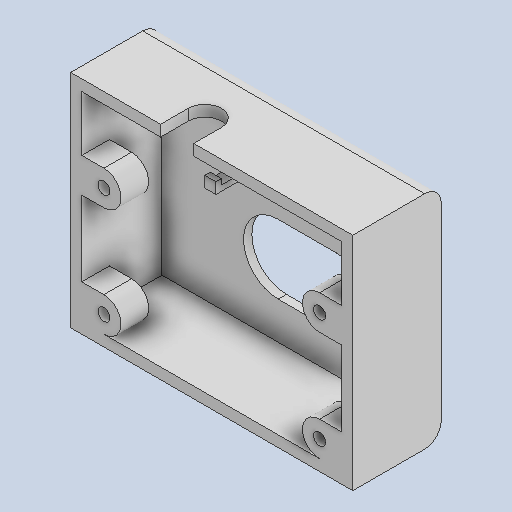
# Autodesk Inventor part: lidarhouse
Saved by Autodesk Inventor 2023.1 (Build 271208000, 208)
## iProperties
Created: 2023-03-22
Part Number: lidarhouse
Material: Generic
Document SubType Name: Modeling
Designer: liaar
Density: 1 g/cm^3
Appearance: Default
Author: liaar
Autodesk Inventor part; units mm, degrees
sketch "Sketch1" plane through (0, 0, 0) normal (0, 0, 1) x (1, 0, 0)
  line L0 (0, 0) -> (51, 0)
  line L1 (51, 0) -> (51, 40)
  line L2 (51, 40) -> (0, 40)
  line L3 (0, 40) -> (0, 0)
  dimension "d0" = 40
  dimension "d1" = 51
  constraints: 8 end point, 2 parallel, 1 horizontal, 1 perpendicular
  measures "d0" distance of L0.end L1.end
  measures "d1" distance of L1.end L2.end
extrude "Extrusion1" add sketch "Sketch1" along normal blind 16
sketch "Sketch2" plane through (0, 0, 16) normal (0, 0, 1) x (1, 0, 0)
  line L0 (2, 38) -> (49, 38)
  line L1 (49, 38) -> (49, 2)
  line L2 (49, 2) -> (2, 2)
  line L3 (2, 2) -> (2, 38)
  line L4 (51, 40) -> (0, 40) projected
  line L5 (0, 40) -> (0, 0) projected
  line L6 (51, 0) -> (51, 40) projected
  line L7 (0, 0) -> (51, 0) projected
  dimension "d4" = 2
  dimension "d5" = 2
  dimension "d6" = 2
  dimension "d7" = 2
  constraints: 8 end point, 2 parallel, 1 horizontal, 1 perpendicular
  measures "d4" distance between parallel lines of L4 L0
  measures "d5" distance between parallel lines of L5 L3
  measures "d6" distance between parallel lines of L6 L1
  measures "d7" distance between parallel lines of L7 L2
extrude "Extrusion2" cut sketch "Sketch2" against normal blind 14.5 contours L0 L1 L2 L3
fillet "Fillet1" radius 3 2 edges at (25.5, 40, 0) (25.5, 0, 0)
sketch "Sketch3" plane through (0, 0, 0) normal (0, 0, -1) x (-1, 0, 0)
  line L0 (-51, 3) -> (-51, 37) projected
  line L1 (0, 37) -> (0, 3) projected
  line L2 (-51, 37) -> (0, 37) projected
  line L3 (0, 3) -> (-51, 3) projected
  circle A0 centre (-33.5, 15) radius 6.25
  circle A1 centre (-23, 15) radius 6.25
  line L4 (-33.5, 21.25) -> (-23, 21.25)
  line L5 (-33.5, 8.75) -> (-23, 8.75)
  line L6 (0, 40) -> (-51, 40) projected
  point P0 (0, 0)
  point P1 (-28.25, 21.25)
  dimension "d49" = 12.5
  dimension "d51" = 10.5
  dimension "d52" = 12.5
  dimension "d54" = 17.5
  dimension "d55" = 22.75
  dimension "d58" = 25
  constraints: 4 end point, 4 point on circle, 4 tangent, 2 centre point, 1 horizontal alignment, 1 midpoint
  measures "d49" diameter of A0
  measures "d51" distance of A0.centre A1.centre
  measures "d52" diameter of A1
  measures "d54" distance from line of L0 A0.centre
  measures "d55" distance from line of L0 point (-28.25, 21.25)
  measures "d58" distance from line of L6 A0.centre
extrude "Extrusion3" cut sketch "Sketch3" against normal blind 14 contours A0 A1 | L4 A1 A0 | A0 A1 L5 | A1 A0 | A0 A1
sketch "Sketch4" plane through (0, 40, 16) normal (0, 1, 0) x (1, 0, 0)
  line L0 (35.25, 0) -> (21.25, 0)
  line L1 (21.25, 0) -> (21.25, 8)
  line L2 (21.25, 8) -> (35.25, 8)
  line L3 (35.25, 8) -> (35.25, 0)
  line L4 (51, 0) -> (0, 0) projected
  line L5 (0, 13) -> (0, 0) projected
  line L6 (51, 13) -> (51, 0) projected
  point P0 (0, 16)
  dimension "d18" = 14
  dimension "d19" = 8
  dimension "d20" = 21.25
  dimension "d21" = 15.75
  constraints: 8 end point, 2 parallel, 1 collinear, 1 horizontal, 1 perpendicular
  measures "d18" distance of L0.start L0.end
  measures "d19" distance of L0.end L1.end
  measures "d20" distance between parallel lines of L5 L1
  measures "d21" distance between parallel lines of L6 L3
ref_plane "Work Plane1" through (0, 0, 16) normal (0, 0, 1) x (1, 0, 0)
sketch "Sketch5" plane through (0, 0, 16) normal (0, 0, 1) x (1, 0, 0)
  circle A0 centre (6, 24.9) radius 3.1
  line L0 (49, 38) -> (49, 2) projected
  line L1 (6, 28) -> (2, 28)
  line L2 (6, 21.8) -> (2, 21.8)
  circle A1 centre (6, 24.9) radius 1.1
  line L3 (2, 2) -> (2, 38) projected
  line L4 (25.5, 34) -> (25.5, 3) construction
  line L5 (0, 3) -> (51, 3) construction
  line L6 (2, 2) -> (2, 38) construction
  line L7 (49, 38) -> (49, 2) construction
  circle A2 centre (6, 5.1) radius 3.1
  line L8 (6, 2) -> (2, 2)
  line L9 (6, 8.2) -> (2, 8.2)
  circle A3 centre (6, 5.1) radius 1.1
  line L10 (2, 38) -> (2, 2)
  line L11 (2, 38) -> (2, 2) construction
  circle A4 centre (45, 24.9) radius 3.1
  line L12 (45, 28) -> (49, 28)
  line L13 (45, 21.8) -> (49, 21.8)
  circle A5 centre (45, 24.9) radius 1.1
  line L14 (49, 2) -> (49, 38)
  line L15 (51, 3) -> (0, 3) construction
  line L16 (49, 2) -> (49, 38) construction
  line L17 (49, 38) -> (49, 2)
  line L18 (49, 38) -> (49, 2) construction
  line L19 (45, 8.2) -> (49, 8.2)
  circle A6 centre (45, 5.1) radius 3.1
  line L20 (45, 2) -> (49, 2)
  circle A7 centre (45, 5.1) radius 1.1
  line L21 (2, 38) -> (49, 38) projected
  line L22 (49, 2) -> (2, 2) projected
  point P0 (0, 0)
  point P1 (4, 28)
  point P2 (4, 2)
  point P3 (47, 28)
  point P4 (47, 2)
  point P5 (49, 8.2)
  point P6 (2, 2)
  point P7 (2, 8.2)
  point P8 (25.5, 38)
  dimension "d28" = 6.2
  dimension "d30" = 4
  dimension "d31" = 2.2
  dimension "d61" = 19.8
  dimension "d62" = 6.2
  constraints: 32 end point, 20 symmetric about line, 9 point on line, 8 centre point, 8 point on circle, 4 coincident, 2 horizontal, 2 midpoint, 2 tangent, 1 collinear, 5 other
  measures "d28" diameter of A0
  measures "d30" distance of L1.start L1.end
  measures "d31" diameter of A1
  measures "d61" distance of A2.centre A0.centre
  measures "d62" diameter of A2
extrude "Extrusion5" add sketch "Sketch5" against normal blind 5 contours A0 | A0 L2 L3 L1 | L9 A2 L8 L3 | A2 | L0 L13 A4 L12 | A4 | A6 | A6 L19 L0 L20
sketch "Sketch6" plane through (0, 0, 11) normal (0, 0, -1) x (-1, 0, 0)
  circle A0 centre (-45, 24.9) radius 1.1 projected
  line L0 (-45, 22.5906) -> (-47, 23.7453)
  line L1 (-47, 23.7453) -> (-47, 26.0547)
  line L2 (-47, 26.0547) -> (-45, 27.2094)
  line L3 (-45, 27.2094) -> (-43, 26.0547)
  line L4 (-43, 26.0547) -> (-43, 23.7453)
  line L5 (-43, 23.7453) -> (-45, 22.5906)
  arc A1 (-6, 28) -> (-6, 21.8) centre (-6, 24.9) ccw projected
  line L6 (-6, 22.5906) -> (-8, 23.7453)
  line L7 (-8, 23.7453) -> (-8, 26.0547)
  line L8 (-8, 26.0547) -> (-6, 27.2094)
  line L9 (-6, 27.2094) -> (-4, 26.0547)
  line L10 (-4, 26.0547) -> (-4, 23.7453)
  line L11 (-4, 23.7453) -> (-6, 22.5906)
  circle A2 centre (-6, 5.1) radius 1.1 projected
  line L12 (-6, 2.7906) -> (-8, 3.9453)
  line L13 (-8, 3.9453) -> (-8, 6.2547)
  line L14 (-8, 6.2547) -> (-6, 7.4094)
  line L15 (-6, 7.4094) -> (-4, 6.2547)
  line L16 (-4, 6.2547) -> (-4, 3.9453)
  line L17 (-4, 3.9453) -> (-6, 2.7906)
  arc A3 (-45, 2) -> (-45, 8.2) centre (-45, 5.1) ccw projected
  line L18 (-45, 2.7906) -> (-47, 3.9453)
  line L19 (-47, 3.9453) -> (-47, 6.2547)
  line L20 (-47, 6.2547) -> (-45, 7.4094)
  line L21 (-45, 7.4094) -> (-43, 6.2547)
  line L22 (-43, 6.2547) -> (-43, 3.9453)
  line L23 (-43, 3.9453) -> (-45, 2.7906)
  circle A4 centre (-45, 5.1) radius 1.1 projected
  circle A5 centre (-6, 24.9) radius 1.1 projected
  point P0 (0, 0)
  point P1 (-6, 38)
  point P2 (-6, 5.1)
  point P3 (-45, 5.1)
  dimension "d45" = 4
  constraints: 48 end point, 4 coincident, 4 vertical alignment, 3 equal length, 52 other
  measures "d45" distance between parallel lines of L3 L0
extrude "Extrusion6" cut sketch "Sketch6" against normal blind 1.7
ref_plane "Work Plane2" through (22.25, 40, 4.75) normal (0, 0, 1) x (1, 0, 0)
sketch "Sketch10" plane through (0, 40, 16) normal (0, 1, 0) x (1, 0, 0)
  line L0 (45, 0) -> (6, 0) projected
  line L1 (16.25, 0) -> (22.25, 0)
  line L2 (22.25, 0) -> (22.25, 5)
  line L3 (22.25, 5) -> (16.25, 5)
  line L4 (16.25, 5) -> (16.25, 0)
  circle A0 centre (19.25, 5) radius 3
  line L5 (0, 13) -> (0, 0) projected
  point P0 (0, 16)
  point P1 (16.25, 5)
  point P2 (22.25, 0)
  dimension "d65" = 16.25
  dimension "d66" = 6
  dimension "d67" = 5
  constraints: 8 end point, 2 parallel, 1 centre point, 1 horizontal, 1 midpoint, 1 perpendicular, 1 point on line, 1 tangent
  measures "d65" distance between parallel lines of L5 L4
  measures "d66" diameter of A0
  measures "d67" distance from line of L0 A0.centre
extrude "Extrusion9" cut sketch "Sketch10" against normal blind 2
ref_plane "Work Plane4" through (22.25, 40, 11) normal (-1, 0, 0) x (0, 0, 1)
sketch "Sketch12" plane through (22.25, 40, 11) normal (-1, 0, 0) x (0, 0, 1)
  line L0 (5, -2) -> (-9.5, -2) projected
  line L1 (-2.5, -7) -> (3, -7)
  line L2 (3, -7) -> (3, -8)
  arc A0 (-8.5, -2) -> (-2.5, -8) centre (-2.5, -2) ccw
  line L3 (3, -8) -> (-2.5, -8)
  arc A1 (-7.5, -2) -> (-2.5, -7) centre (-2.5, -2) ccw
  line L4 (3, -7) -> (2, -7)
  line L5 (2, -7) -> (2, -6)
  line L6 (2, -6) -> (3, -6)
  line L7 (3, -6) -> (3, -7)
  point P0 (-11, -40)
  point P1 (-3, -2)
  point P2 (3.5, -2)
  point P3 (2, -7)
  dimension "d73" = 1
  dimension "d74" = 5
  dimension "d77" = 1
  dimension "d78" = 1
  dimension "d79" = 1
  dimension "d80" = 4.5
  dimension "d81" = 5
  constraints: 14 end point, 4 point on circle, 3 parallel, 3 point on line, 2 centre point, 2 horizontal, 2 tangent, 1 concentric, 1 perpendicular, 1 vertical
  measures "d73" distance of L1.end L2.end
  measures "d74" distance between parallel lines of L0 L1
  measures "d77" distance of A1.start A0.start
  measures "d78" distance of L6.end L1.end
  measures "d79" distance of L5.end L6.end
  measures "d80" distance of point (-3, -2) A1.start
  measures "d81" distance from line of point (-3, -2) L5
extrude "Extrusion10" add sketch "Sketch12" against normal blind 2
body "Solid1"
